Autodesk Inventor part; units mm, degrees
(part 2 of 2)
sketch "Sketch9" plane through (0, 4.7752, 0) normal (0, 1, 0) x (1, 0, 0)
  line L0 (-19.05, 266.7) -> (-234.95, 76.2) construction
  line L1 (-234.95, 266.7) -> (-19.05, 76.2) construction
  line L2 (0, 339.725) -> (0, 3.175) projected
  circle A0 centre (-12.7, 171.45) radius 2.8067 projected
  line L3 (-3.175, 0) -> (-25.4, 0) projected
  line L4 (-127, 171.45) -> (-127, 146.05)
  line L5 (-127, 171.45) -> (-101.6, 171.45)
  line L6 (-103.8451, 169.2049) -> (-124.7549, 148.2951)
  line L7 (-127, 171.45) -> (-127, 196.85)
  line L8 (-127, 171.45) -> (-152.4, 171.45)
  line L9 (-129.2451, 148.2951) -> (-150.1549, 169.2049)
  line L10 (-150.1549, 173.6951) -> (-129.2451, 194.6049)
  line L11 (-124.7549, 194.6049) -> (-103.8451, 173.6951)
  line L12 (-90.9194, 164.1701) -> (-119.7201, 135.3694)
  line L13 (-101.6, 171.45) -> (-19.05, 171.45)
  line L14 (-127, 146.05) -> (-127, 76.2)
  line L15 (-101.6, 171.45) -> (-127, 146.05)
  line L16 (-127, 196.85) -> (-101.6, 171.45)
  line L17 (-77.449, 159.6799) -> (-115.2299, 121.899)
  line L18 (-54.9984, 164.1701) -> (-119.7201, 99.4484)
  line L19 (-41.528, 159.6799) -> (-115.2299, 85.978)
  line L20 (-24.4701, 158.7774) -> (-101.6274, 81.6201)
  line L21 (-19.9799, 145.307) -> (-88.157, 77.1299)
  line L22 (-24.4701, 122.8564) -> (-65.7064, 81.6201)
  line L23 (-19.9799, 109.386) -> (-52.236, 77.1299)
  line L24 (-88.6744, 165.1) -> (-79.6941, 165.1)
  line L25 (-52.7533, 165.1) -> (-43.7731, 165.1)
  line L26 (-120.65, 133.1244) -> (-120.65, 124.1441)
  line L27 (-120.65, 97.2033) -> (-120.65, 88.2231)
  line L28 (-24.4701, 86.9353) -> (-29.7853, 81.6201)
  line L29 (-19.05, 79.375) -> (-19.05, 84.6903)
  line L30 (-19.05, 111.631) -> (-19.05, 120.6113)
  line L31 (-63.4613, 76.2) -> (-54.481, 76.2)
  line L32 (-27.5403, 76.2) -> (-22.225, 76.2)
  line L33 (-19.05, 147.5521) -> (-19.05, 156.5323)
  line L34 (-99.3823, 76.2) -> (-90.4021, 76.2)
  arc A1 (-22.225, 76.2) -> (-19.05, 79.375) centre (-22.225, 79.375) ccw
  arc A2 (-19.05, 84.6903) -> (-24.4701, 86.9353) centre (-22.225, 84.6903) ccw
  arc A3 (-29.7853, 81.6201) -> (-27.5403, 76.2) centre (-27.5403, 79.375) ccw
  arc A4 (-54.481, 76.2) -> (-52.236, 77.1299) centre (-54.481, 79.375) ccw
  arc A5 (-19.9799, 109.386) -> (-19.05, 111.631) centre (-22.225, 111.631) ccw
  arc A6 (-19.05, 120.6113) -> (-24.4701, 122.8564) centre (-22.225, 120.6113) ccw
  arc A7 (-65.7064, 81.6201) -> (-63.4613, 76.2) centre (-63.4613, 79.375) ccw
  arc A8 (-90.4021, 76.2) -> (-88.157, 77.1299) centre (-90.4021, 79.375) ccw
  arc A9 (-101.6274, 81.6201) -> (-99.3823, 76.2) centre (-99.3823, 79.375) ccw
  arc A10 (-19.05, 156.5323) -> (-24.4701, 158.7774) centre (-22.225, 156.5323) ccw
  arc A11 (-19.9799, 145.307) -> (-19.05, 147.5521) centre (-22.225, 147.5521) ccw
  arc A12 (-41.528, 159.6799) -> (-43.7731, 165.1) centre (-43.7731, 161.925) ccw
  arc A13 (-52.7533, 165.1) -> (-54.9984, 164.1701) centre (-52.7533, 161.925) ccw
  arc A14 (-119.7201, 99.4484) -> (-120.65, 97.2033) centre (-117.475, 97.2033) ccw
  arc A15 (-120.65, 88.2231) -> (-115.2299, 85.978) centre (-117.475, 88.2231) ccw
  arc A16 (-120.65, 124.1441) -> (-115.2299, 121.899) centre (-117.475, 124.1441) ccw
  arc A17 (-119.7201, 135.3694) -> (-120.65, 133.1244) centre (-117.475, 133.1244) ccw
  arc A18 (-88.6744, 165.1) -> (-90.9194, 164.1701) centre (-88.6744, 161.925) ccw
  arc A19 (-77.449, 159.6799) -> (-79.6941, 165.1) centre (-79.6941, 161.925) ccw
  arc A20 (-129.2451, 148.2951) -> (-124.7549, 148.2951) centre (-127, 150.5401) ccw
  arc A21 (-103.8451, 169.2049) -> (-103.8451, 173.6951) centre (-106.0901, 171.45) ccw
  arc A22 (-124.7549, 194.6049) -> (-129.2451, 194.6049) centre (-127, 192.3599) ccw
  arc A23 (-150.1549, 173.6951) -> (-150.1549, 169.2049) centre (-147.9099, 171.45) ccw
  circle A24 centre (-12.7, 171.45) radius 2.8067
  line L35 (-127, 171.45) -> (-127, 196.85)
  line L36 (-103.8451, 173.6951) -> (-124.7549, 194.6049)
  line L37 (-90.9194, 178.7299) -> (-119.7201, 207.5306)
  line L38 (-127, 196.85) -> (-127, 266.7)
  line L39 (-101.6, 171.45) -> (-127, 196.85)
  line L40 (-77.449, 183.2201) -> (-115.2299, 221.001)
  line L41 (-54.9984, 178.7299) -> (-119.7201, 243.4516)
  line L42 (-41.528, 183.2201) -> (-115.2299, 256.922)
  line L43 (-24.4701, 184.1226) -> (-101.6274, 261.2799)
  line L44 (-19.9799, 197.593) -> (-88.157, 265.7701)
  line L45 (-24.4701, 220.0436) -> (-65.7064, 261.2799)
  line L46 (-19.9799, 233.514) -> (-52.236, 265.7701)
  line L47 (-88.6744, 177.8) -> (-79.6941, 177.8)
  line L48 (-52.7533, 177.8) -> (-43.7731, 177.8)
  line L49 (-120.65, 209.7756) -> (-120.65, 218.7559)
  line L50 (-120.65, 245.6967) -> (-120.65, 254.6769)
  line L51 (-24.4701, 255.9647) -> (-29.7853, 261.2799)
  line L52 (-19.05, 263.525) -> (-19.05, 258.2097)
  line L53 (-19.05, 231.269) -> (-19.05, 222.2887)
  line L54 (-63.4613, 266.7) -> (-54.481, 266.7)
  line L55 (-27.5403, 266.7) -> (-22.225, 266.7)
  line L56 (-19.05, 195.3479) -> (-19.05, 186.3677)
  line L57 (-99.3823, 266.7) -> (-90.4021, 266.7)
  arc A25 (-19.05, 263.525) -> (-22.225, 266.7) centre (-22.225, 263.525) ccw
  arc A26 (-24.4701, 255.9647) -> (-19.05, 258.2097) centre (-22.225, 258.2097) ccw
  arc A27 (-27.5403, 266.7) -> (-29.7853, 261.2799) centre (-27.5403, 263.525) ccw
  arc A28 (-52.236, 265.7701) -> (-54.481, 266.7) centre (-54.481, 263.525) ccw
  arc A29 (-19.05, 231.269) -> (-19.9799, 233.514) centre (-22.225, 231.269) ccw
  arc A30 (-24.4701, 220.0436) -> (-19.05, 222.2887) centre (-22.225, 222.2887) ccw
  arc A31 (-63.4613, 266.7) -> (-65.7064, 261.2799) centre (-63.4613, 263.525) ccw
  arc A32 (-88.157, 265.7701) -> (-90.4021, 266.7) centre (-90.4021, 263.525) ccw
  arc A33 (-99.3823, 266.7) -> (-101.6274, 261.2799) centre (-99.3823, 263.525) ccw
  arc A34 (-24.4701, 184.1226) -> (-19.05, 186.3677) centre (-22.225, 186.3677) ccw
  arc A35 (-19.05, 195.3479) -> (-19.9799, 197.593) centre (-22.225, 195.3479) ccw
  arc A36 (-43.7731, 177.8) -> (-41.528, 183.2201) centre (-43.7731, 180.975) ccw
  arc A37 (-54.9984, 178.7299) -> (-52.7533, 177.8) centre (-52.7533, 180.975) ccw
  arc A38 (-120.65, 245.6967) -> (-119.7201, 243.4516) centre (-117.475, 245.6967) ccw
  arc A39 (-115.2299, 256.922) -> (-120.65, 254.6769) centre (-117.475, 254.6769) ccw
  arc A40 (-115.2299, 221.001) -> (-120.65, 218.7559) centre (-117.475, 218.7559) ccw
  arc A41 (-120.65, 209.7756) -> (-119.7201, 207.5306) centre (-117.475, 209.7756) ccw
  arc A42 (-90.9194, 178.7299) -> (-88.6744, 177.8) centre (-88.6744, 180.975) ccw
  arc A43 (-79.6941, 177.8) -> (-77.449, 183.2201) centre (-79.6941, 180.975) ccw
  arc A44 (-124.7549, 194.6049) -> (-129.2451, 194.6049) centre (-127, 192.3599) ccw
  arc A45 (-103.8451, 169.2049) -> (-103.8451, 173.6951) centre (-106.0901, 171.45) ccw
  line L58 (-234.95, 266.7) -> (-19.05, 76.2) construction
  line L59 (-19.05, 266.7) -> (-234.95, 76.2) construction
  line L60 (-254, 339.725) -> (-254, 3.175)
  line L61 (-150.1549, 169.2049) -> (-129.2451, 148.2951)
  line L62 (-129.2451, 194.6049) -> (-150.1549, 173.6951)
  line L63 (-163.0806, 164.1701) -> (-134.2799, 135.3694)
  line L64 (-152.4, 171.45) -> (-127, 146.05)
  line L65 (-127, 196.85) -> (-152.4, 171.45)
  line L66 (-176.551, 159.6799) -> (-138.7701, 121.899)
  line L67 (-199.0016, 164.1701) -> (-134.2799, 99.4484)
  line L68 (-212.472, 159.6799) -> (-138.7701, 85.978)
  line L69 (-229.5299, 158.7774) -> (-152.3726, 81.6201)
  line L70 (-234.0201, 145.307) -> (-165.843, 77.1299)
  line L71 (-229.5299, 122.8564) -> (-188.2936, 81.6201)
  line L72 (-234.0201, 109.386) -> (-201.764, 77.1299)
  line L73 (-165.3256, 165.1) -> (-174.3059, 165.1)
  line L74 (-201.2467, 165.1) -> (-210.2269, 165.1)
  line L75 (-133.35, 133.1244) -> (-133.35, 124.1441)
  line L76 (-133.35, 97.2033) -> (-133.35, 88.2231)
  line L77 (-229.5299, 86.9353) -> (-224.2147, 81.6201)
  line L78 (-234.95, 79.375) -> (-234.95, 84.6903)
  line L79 (-234.95, 111.631) -> (-234.95, 120.6113)
  line L80 (-190.5387, 76.2) -> (-199.519, 76.2)
  line L81 (-226.4597, 76.2) -> (-231.775, 76.2)
  line L82 (-234.95, 147.5521) -> (-234.95, 156.5323)
  line L83 (-154.6177, 76.2) -> (-163.5979, 76.2)
  arc A46 (-234.95, 79.375) -> (-231.775, 76.2) centre (-231.775, 79.375) ccw
  arc A47 (-229.5299, 86.9353) -> (-234.95, 84.6903) centre (-231.775, 84.6903) ccw
  arc A48 (-226.4597, 76.2) -> (-224.2147, 81.6201) centre (-226.4597, 79.375) ccw
  arc A49 (-201.764, 77.1299) -> (-199.519, 76.2) centre (-199.519, 79.375) ccw
  arc A50 (-234.95, 111.631) -> (-234.0201, 109.386) centre (-231.775, 111.631) ccw
  arc A51 (-229.5299, 122.8564) -> (-234.95, 120.6113) centre (-231.775, 120.6113) ccw
  arc A52 (-190.5387, 76.2) -> (-188.2936, 81.6201) centre (-190.5387, 79.375) ccw
  arc A53 (-165.843, 77.1299) -> (-163.5979, 76.2) centre (-163.5979, 79.375) ccw
  arc A54 (-154.6177, 76.2) -> (-152.3726, 81.6201) centre (-154.6177, 79.375) ccw
  arc A55 (-229.5299, 158.7774) -> (-234.95, 156.5323) centre (-231.775, 156.5323) ccw
  arc A56 (-234.95, 147.5521) -> (-234.0201, 145.307) centre (-231.775, 147.5521) ccw
  arc A57 (-210.2269, 165.1) -> (-212.472, 159.6799) centre (-210.2269, 161.925) ccw
  arc A58 (-199.0016, 164.1701) -> (-201.2467, 165.1) centre (-201.2467, 161.925) ccw
  arc A59 (-133.35, 97.2033) -> (-134.2799, 99.4484) centre (-136.525, 97.2033) ccw
  arc A60 (-138.7701, 85.978) -> (-133.35, 88.2231) centre (-136.525, 88.2231) ccw
  arc A61 (-138.7701, 121.899) -> (-133.35, 124.1441) centre (-136.525, 124.1441) ccw
  arc A62 (-133.35, 133.1244) -> (-134.2799, 135.3694) centre (-136.525, 133.1244) ccw
  arc A63 (-163.0806, 164.1701) -> (-165.3256, 165.1) centre (-165.3256, 161.925) ccw
  arc A64 (-174.3059, 165.1) -> (-176.551, 159.6799) centre (-174.3059, 161.925) ccw
  line L84 (-234.0201, 233.514) -> (-201.764, 265.7701)
  line L85 (-229.5299, 220.0436) -> (-188.2936, 261.2799)
  line L86 (-234.0201, 197.593) -> (-165.843, 265.7701)
  line L87 (-229.5299, 184.1226) -> (-152.3726, 261.2799)
  line L88 (-212.472, 183.2201) -> (-138.7701, 256.922)
  line L89 (-199.0016, 178.7299) -> (-134.2799, 243.4516)
  line L90 (-176.551, 183.2201) -> (-138.7701, 221.001)
  line L91 (-163.0806, 178.7299) -> (-134.2799, 207.5306)
  line L92 (-150.1549, 173.6951) -> (-129.2451, 194.6049)
  line L93 (-152.4, 171.45) -> (-127, 196.85)
  line L94 (-229.5299, 255.9647) -> (-224.2147, 261.2799)
  line L95 (-226.4597, 266.7) -> (-231.775, 266.7)
  arc A65 (-224.2147, 261.2799) -> (-226.4597, 266.7) centre (-226.4597, 263.525) ccw
  arc A66 (-163.5979, 266.7) -> (-165.843, 265.7701) centre (-163.5979, 263.525) ccw
  arc A67 (-188.2936, 261.2799) -> (-190.5387, 266.7) centre (-190.5387, 263.525) ccw
  line L96 (-190.5387, 266.7) -> (-199.519, 266.7)
  arc A68 (-199.519, 266.7) -> (-201.764, 265.7701) centre (-199.519, 263.525) ccw
  line L97 (-133.35, 209.7756) -> (-133.35, 218.7559)
  line L98 (-133.35, 245.6967) -> (-133.35, 254.6769)
  line L99 (-154.6177, 266.7) -> (-163.5979, 266.7)
  arc A69 (-152.3726, 261.2799) -> (-154.6177, 266.7) centre (-154.6177, 263.525) ccw
  arc A70 (-133.35, 254.6769) -> (-138.7701, 256.922) centre (-136.525, 254.6769) ccw
  arc A71 (-134.2799, 243.4516) -> (-133.35, 245.6967) centre (-136.525, 245.6967) ccw
  arc A72 (-133.35, 218.7559) -> (-138.7701, 221.001) centre (-136.525, 218.7559) ccw
  arc A73 (-134.2799, 207.5306) -> (-133.35, 209.7756) centre (-136.525, 209.7756) ccw
  arc A74 (-165.3256, 177.8) -> (-163.0806, 178.7299) centre (-165.3256, 180.975) ccw
  line L100 (-165.3256, 177.8) -> (-174.3059, 177.8)
  arc A75 (-176.551, 183.2201) -> (-174.3059, 177.8) centre (-174.3059, 180.975) ccw
  line L101 (-201.2467, 177.8) -> (-210.2269, 177.8)
  line L102 (-234.95, 231.269) -> (-234.95, 222.2887)
  line L103 (-234.95, 195.3479) -> (-234.95, 186.3677)
  arc A76 (-234.0201, 233.514) -> (-234.95, 231.269) centre (-231.775, 231.269) ccw
  arc A77 (-234.95, 222.2887) -> (-229.5299, 220.0436) centre (-231.775, 222.2887) ccw
  arc A78 (-234.95, 186.3677) -> (-229.5299, 184.1226) centre (-231.775, 186.3677) ccw
  arc A79 (-212.472, 183.2201) -> (-210.2269, 177.8) centre (-210.2269, 180.975) ccw
  arc A80 (-234.0201, 197.593) -> (-234.95, 195.3479) centre (-231.775, 195.3479) ccw
  arc A81 (-201.2467, 177.8) -> (-199.0016, 178.7299) centre (-201.2467, 180.975) ccw
  arc A82 (-234.95, 258.2097) -> (-229.5299, 255.9647) centre (-231.775, 258.2097) ccw
  line L104 (-234.95, 263.525) -> (-234.95, 258.2097)
  arc A83 (-231.775, 266.7) -> (-234.95, 263.525) centre (-231.775, 263.525) ccw
  point P0 (0, 0)
  point P1 (-127, 171.45)
  dimension "d224" = 190.5
  dimension "d225" = 215.9
  dimension "d226" = 114.3
  dimension "d227" = 171.45
  dimension "d228" = 25.4
  dimension "d229" = 25.4
  dimension "d230" = 25.4
  dimension "d231" = 25.4
  dimension "d233" = 12.7
  dimension "d244" = 12.7
  dimension "d249" = 12.7
  dimension "d250" = 12.7
  dimension "d251" = 12.7
  dimension "d252" = 12.7
  dimension "d253" = 12.7
  dimension "d254" = 12.7
  dimension "d255" = 12.7
  dimension "d256" = 12.7
  dimension "d257" = 3.175
  constraints: 206 end point, 188 symmetric about line, 164 point on circle, 83 centre point, 46 tangent, 22 equal radius, 17 point on line, 14 parallel, 2 midpoint, 1 perpendicular, 1 vertical, 60 other
  measures "d224" distance of L1.end L0.start
  measures "d225" distance of L0.start L1.start
  measures "d226" distance of A0.centre point (-127, 171.45)
  measures "d227" distance from line of L3 L4.start
  measures "d228" distance of L4.start L4.end
  measures "d229" distance of L4.start L5.end
  measures "d230" distance of L4.start L7.end
  measures "d231" distance of L4.start L8.end
  measures "d233" distance between parallel lines of L6 L12
  measures "d244" distance between parallel lines of L12 L15
  measures "d249" distance between parallel lines of L12 L17
  measures "d250" distance between parallel lines of L17 L18
  measures "d251" distance between parallel lines of L18 L19
  measures "d252" distance between parallel lines of L19 L20
  measures "d253" distance between parallel lines of L20 L21
  measures "d254" distance between parallel lines of L21 L22
  measures "d255" distance between parallel lines of L22 L23
  measures "d256" distance between parallel lines of L23 L28
  measures "d257" radius of A1
extrude "Extrusion8" cut sketch "Sketch9" against normal through all contours L5 A21 L6 A20 L4 | L7 A22 L11 A21 L5 | L8 A23 L10 A22 L7 | L4 A20 L9 A23 L8 | A18 L24 A19 L17 A16 L26 A17 L12 | A13 L25 A12 L19 A15 L27 A14 L18 | A10 L33 A11 L21 A8 L34 A9 L20 | A6 L30 A5 L23 A4 L31 A7 L22 | A2 L29 A1 L32 A3 L28 | L37 A41 L49 A40 L40 A43 L47 A42 | L41 A38 L50 A39 L42 A36 L48 A37 | L43 A33 L57 A32 L44 A35 L56 A34 | L45 A31 L54 A28 L46 A29 L53 A30 | L51 A27 L55 A25 L52 A26 | L63 A62 L75 A61 L66 A64 L73 A63 | L67 A59 L76 A60 L68 A57 L74 A58 | L69 A54 L83 A53 L70 A56 L82 A55 | L71 A52 L80 A49 L72 A50 L79 A51 | L77 A48 L81 A46 L78 A47 | L84 A68 L96 A67 L85 A77 L102 A76 | L86 A66 L99 A69 L87 A78 L103 A80 | L88 A70 L98 A71 L89 A81 L101 A79 | L90 A72 L97 A73 L91 A74 L100 A75 | A82 L104 A83 L95 A65 L94
sketch "Sketch10" plane through (0, 4.7752, 0) normal (0, 1, 0) x (1, 0, 0)
  line L0 (-254, 76.2) -> (-431.8, 76.2)
  line L1 (-431.8, 76.2) -> (-431.8, 266.7)
  line L2 (-431.8, 266.7) -> (-254, 266.7)
  line L3 (-254, 266.7) -> (-254, 76.2)
  line L4 (-254, 76.2) -> (-431.8, 266.7) construction
  line L5 (-431.8, 76.2) -> (-254, 266.7) construction
  line L6 (-511.175, 514.35) -> (-174.625, 514.35) projected
  line L7 (-685.8, 3.175) -> (-685.8, 339.725) projected
  line L8 (-342.9, 171.45) -> (-317.5, 171.45) construction
  line L9 (-342.9, 171.45) -> (-393.7, 171.45) construction
  line L10 (-393.7, 158.75) -> (-342.9, 158.75)
  line L11 (-393.7, 184.15) -> (-342.9, 184.15)
  line L12 (-317.5, 184.15) -> (-342.9, 184.15)
  line L13 (-320.675, 184.15) -> (-390.525, 184.15)
  line L14 (-320.675, 158.75) -> (-342.9, 158.75)
  line L15 (-342.9, 158.75) -> (-390.525, 158.75)
  line L16 (-317.5, 171.45) -> (-279.4, 171.45)
  line L17 (-281.6451, 173.6951) -> (-312.0799, 204.1299)
  line L18 (-279.4, 171.45) -> (-207.558, 171.45) construction
  line L19 (-281.6451, 169.2049) -> (-312.0799, 138.7701)
  line L20 (-279.4, 171.45) -> (-207.558, 171.45) construction
  line L21 (-317.5, 155.575) -> (-317.5, 141.0151)
  line L22 (-317.5, 187.325) -> (-317.5, 201.8849)
  line L23 (-393.7, 180.975) -> (-393.7, 161.925)
  arc A0 (-390.525, 184.15) -> (-393.7, 180.975) centre (-390.525, 180.975) ccw
  arc A1 (-320.675, 184.15) -> (-317.5, 187.325) centre (-320.675, 187.325) ccw
  arc A2 (-312.0799, 204.1299) -> (-317.5, 201.8849) centre (-314.325, 201.8849) ccw
  arc A3 (-281.6451, 169.2049) -> (-281.6451, 173.6951) centre (-283.8901, 171.45) ccw
  arc A4 (-317.5, 141.0151) -> (-312.0799, 138.7701) centre (-314.325, 141.0151) ccw
  arc A5 (-317.5, 155.575) -> (-320.675, 158.75) centre (-320.675, 155.575) ccw
  arc A6 (-393.7, 161.925) -> (-390.525, 158.75) centre (-390.525, 161.925) ccw
  point P0 (0, 0)
  point P1 (-317.5, 209.55)
  dimension "d260" = 342.9
  dimension "d261" = 342.9
  dimension "d262" = 190.5
  dimension "d263" = 177.8
  dimension "d264" = 25.4
  dimension "d265" = 50.8
  dimension "d266" = 12.7
  dimension "d267" = 12.7
  dimension "d268" = 12.7
  dimension "d269" = 12.7
  dimension "d270" = 38.1
  dimension "d271" = 135
  dimension "d272" = 135
  dimension "d273" = 3.175
  dimension "d274" = 3.175
  constraints: 44 end point, 14 point on circle, 14 tangent, 7 centre point, 7 point on line, 6 horizontal, 5 equal radius, 2 midpoint, 2 parallel, 2 perpendicular, 1 vertical, 2 other
  measures "d260" distance from line of L6 L8.start
  measures "d261" distance from line of L7 L8.start
  measures "d262" distance of L0.end L1.end
  measures "d263" distance of L1.end L2.end
  measures "d264" distance of L8.start L8.end
  measures "d265" distance of L8.start L9.end
  measures "d266" distance between parallel lines of L9 L10
  measures "d267" distance between parallel lines of L9 L11
  measures "d268" distance between parallel lines of L8 L12
  measures "d269" distance between parallel lines of L8 L14
  measures "d270" distance of L8.end L16.end
  measures "d271" angle of L18 L17
  measures "d272" angle of L19 L20
  measures "d273" radius of A0
  measures "d274" radius of A2
extrude "Extrusion9" cut sketch "Sketch10" against normal through all contours A6 L23 A0 L11 L12 A1 L22 A2 L17 A3 L19 A4 L21 A5 L14 L10
ref_plane "Work Plane1" through (-342.9, 0, -3.175) normal (1, 0, 0) x (0, 0, -1)
mirror "Mirror1" about plane through (-342.9, 0, -3.175) normal (1, 0, 0) of "Extrusion8"
equation "\"d21\" = d22"
equation "\"d22\" = d19"
equation "\"d51\" = d50"
body "Solid1"
